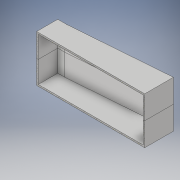
# Autodesk Inventor part: EnclosureTop
Saved by Autodesk Inventor 2019 (Build 230136000, 136)
## iProperties
Created: 2018-11-13
Part Number: EnclosureTop
Material: Generic
Document SubType Name: Modeling
Designer: cvill
Density: 1 g/cm^3
Appearance: Default
Author: cvill
Autodesk Inventor part; units mm, degrees
ref_plane "YZ Plane" through (0, 0, 0) normal (1, 0, 0) x (0, 1, 0)
ref_plane "XZ Plane" through (0, 0, 0) normal (0, 1, 0) x (-1, 0, 0)
ref_plane "XY Plane" through (0, 0, 0) normal (0, 0, 1) x (1, 0, 0)
sketch "Sketch1" plane through (0, 0, 0) normal (0, 1, 0) x (-1, 0, 0)
  point P0 (0, 0)
sketch "Sketch2" plane through (0, 0, 0) normal (0, 1, 0) x (-1, 0, 0)
  line L0 (0, 0) -> (88.9, 0)
  line L1 (88.9, 0) -> (88.9, -40.64)
  line L2 (88.9, -40.64) -> (82.7769, -40.64)
  line L3 (0, -40.64) -> (0, 0)
  line L4 (0, -40.64) -> (0, -46.99)
  line L5 (0, -46.99) -> (82.7769, -40.64)
  line L6 (88.9, 1.397) -> (0, 1.397)
  line L7 (0, 1.397) -> (-1.397, 1.397)
  line L8 (-1.397, 1.397) -> (-1.397, -42.037)
  line L9 (-1.397, -42.037) -> (-1.397, -47.0972)
  line L10 (-1.397, -47.0972) -> (-1.397, -48.4942)
  line L11 (-1.397, -48.4942) -> (82.7769, -42.037)
  line L12 (82.7769, -42.037) -> (88.9, -42.037)
  line L13 (88.9, -42.037) -> (90.297, -42.037)
  line L14 (90.297, -42.037) -> (90.297, 1.397)
  line L15 (90.297, 1.397) -> (88.9, 1.397)
  dimension "d0" = 88.9
  dimension "d2" = 6.35
  dimension "d6" = 1.397
  dimension "d7" = 43.434
  dimension "d8" = 1.397
  dimension "d9" = 1.397
  constraints: 32 end point, 6 point on line, 5 perpendicular, 4 parallel, 1 horizontal
  measures "d0" distance of L1.end L3.start
  measures "d2" distance of L3.start L4.end
  measures "d6" distance of L6.end L7.end
  measures "d7" distance of L7.end L8.end
  measures "d8" distance of L9.end L10.end
  measures "d9" distance of L12.end L13.end
extrude "Extrusion1" add sketch "Sketch2" along normal blind 36.83
sketch "Sketch3" plane through (0, 36.83, 0) normal (0, 1, 0) x (1, 0, 0)
  point P0 (0, 0)
sketch "Sketch4" plane through (0, 36.83, 0) normal (0, 1, 0) x (1, 0, 0)
  line L0 (-90.297, -1.397) -> (1.397, -1.397) projected
  line L1 (1.397, -1.397) -> (1.397, 48.5083)
  line L2 (-82.7769, 42.037) -> (-90.297, 42.037) projected
  line L3 (1.397, 48.5083) -> (-82.7769, 42.037)
  line L4 (-82.7769, 42.037) -> (-90.297, 42.037)
  line L5 (-90.297, 42.037) -> (-90.297, -1.397) projected
  line L6 (-90.297, 42.037) -> (-90.297, -1.397)
  line L7 (1.397, -1.397) -> (1.397, 48.4942) projected
  line L8 (-90.297, -1.397) -> (1.397, -1.397)
  line L9 (1.397, -1.397) -> (1.397, 48.4942)
  point P0 (0, 0)
  constraints: 12 end point, 3 perpendicular, 1 collinear, 1 vertical
extrude "Extrusion2" add sketch "Sketch4" along normal blind 1.397
sketch "Sketch5" plane through (0, 0, 0) normal (0, -1, 0) x (1, 0, 0)
  line L0 (1.397, -48.4942) -> (-82.7769, -42.037) projected
  line L1 (1.397, -48.4942) -> (-82.7769, -42.037)
  line L2 (-82.7769, -42.037) -> (-90.297, -42.037)
  line L3 (-90.297, 1.397) -> (1.397, 1.397) projected
  line L4 (-90.297, -42.037) -> (-90.297, 1.397)
  line L5 (-90.297, 1.397) -> (1.397, 1.397)
  line L6 (1.397, 1.397) -> (1.397, -48.4942)
  point P0 (0, 0)
  constraints: 10 end point, 2 collinear, 2 perpendicular, 1 horizontal
extrude "Extrusion3" add sketch "Sketch5" along normal blind 1.397
sketch "Sketch6" plane through (-82.7769, -1.397, -42.037) normal (-0.0764875, 0, -0.9970705) x (-0.9970705, 0, 0.0764875)
  point P0 (-79.3191, 1.397)
sketch "Sketch7" plane through (-90.297, 38.227, 1.397) normal (0, 0, 1) x (1, 0, 0)
  line L0 (0, -39.624) -> (0, 0) projected
  line L1 (0, -19.812) -> (91.694, -19.812)
  line L2 (91.694, -39.624) -> (91.694, 0) projected
  point P0 (90.297, -38.227)
  constraints: 2 end point, 2 midpoint
split body "Split1" sketch "Sketch7" result two bodies curves L1 first body at (-26.661, 37.727, -29.7114)
body "Solid2"
body "Solid3"
